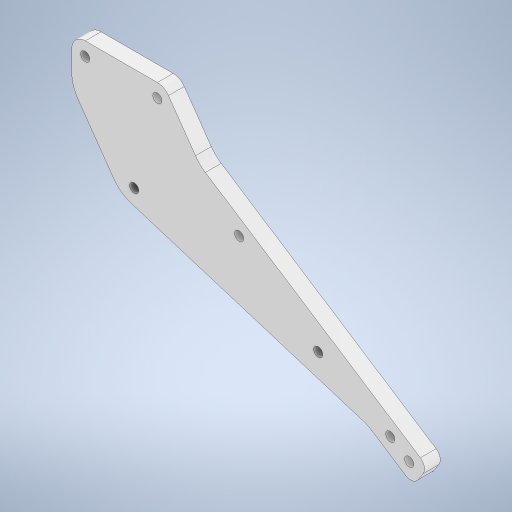
# Autodesk Inventor part: Tibia_V2
Saved by Autodesk Inventor 2024 (Build 280153000, 153)
## iProperties
Created: 2024-06-04
Part Number: Tibia_V2
Material: Generic
Document SubType Name: Modeling
Designer: Hemant
Density: 1 g/cm^3
Appearance: White
Author: Hemant
Autodesk Inventor part; units mm, degrees
ref_plane "YZ Plane" through (0, 0, 0) normal (1, 0, 0) x (0, 1, 0)
ref_plane "XZ Plane" through (0, 0, 0) normal (0, 1, 0) x (-1, 0, 0)
ref_plane "XY Plane" through (0, 0, 0) normal (0, 0, 1) x (1, 0, 0)
sketch "Sketch1" plane through (0, 0, 0) normal (0, 0, 1) x (1, 0, 0)
  line L0 (0, 0) -> (22, 0)
  circle A0 centre (3, -3) radius 1
  circle A1 centre (19, -3) radius 1
  circle A2 centre (19, -3) radius 3
  circle A3 centre (3, -3) radius 3
  line L1 (0, -10) -> (27.5638, -10) construction
  line L2 (22, 0) -> (30.0637, -11.5162) construction
  line L3 (22, 0) -> (36.0586, 0) construction
  line L4 (0, -10) -> (0, -3)
  line L5 (28.3404, -11.1091) -> (21.4575, -1.2793)
  line L6 (0, -10) -> (10.7416, -25.3406)
  circle A4 centre (26.0021, -13) radius 1 construction
  line L7 (28.3404, -11.1091) -> (79, -44.0078)
  line L8 (28.3404, -11.1091) -> (26.0021, -13) construction
  line L9 (26.0021, -13) -> (10.7416, -25.3406) construction
  circle A5 centre (13.8594, -22.8194) radius 1
  line L10 (79, -101.0698) -> (79, 42.0759) construction
  line L11 (79, -44.0078) -> (75.7322, -49.0399)
  circle A6 centre (74.8501, -44.8899) radius 1
  line L12 (75.7322, -49.0399) -> (65.6681, -42.5042)
  circle A7 centre (70.6567, -42.1667) radius 1
  line L13 (65.6681, -42.5042) -> (10.7416, -25.3406)
  circle A8 centre (13.8594, -22.8194) radius 3 construction
  circle A9 centre (26.0021, -13) radius 3 construction
  line L14 (67.4577, -36.7773) -> (-2.3075, -14.9769) construction
  line L15 (-2.3075, -14.9769) -> (-9.5668, -6) construction
  line L16 (90.7322, -58.781) -> (24.0944, -15.5059) construction
  line L17 (24.0944, -15.5059) -> (16.5425, -4.7207) construction
  line L18 (47.0108, -30.388) -> (1.9372, -16.3033) construction
  line L19 (1.9372, -16.3033) -> (12.3526, -7.8807) construction
  line L20 (12.3526, -7.8807) -> (47.0108, -30.388) construction
  line L21 (0, -6) -> (22, -6) construction
  line L22 (-9.5668, -6) -> (17.4383, -6) construction
  line L23 (17.4383, -6) -> (22.4483, -13.155) construction
  line L24 (22.4483, -13.155) -> (6.5898, -25.9792) construction
  line L25 (6.5898, -25.9792) -> (-9.5668, -6) construction
  circle A10 centre (54.6727, -33.8896) radius 1
  circle A11 centre (37.1374, -20.399) radius 1
  circle A12 centre (37.1374, -20.399) radius 3 construction
  point P0 (19, 0)
  point P1 (3, 0)
  dimension "d0" = 22
  dimension "d1" = 2
  dimension "d2" = 2
  dimension "d3" = 16
  dimension "d4" = 3
  dimension "d5" = 3
  dimension "d6" = 2
  dimension "d7" = 2
  dimension "d8" = 10
  dimension "d9" = 55
  dimension "d10" = 2
  dimension "d11" = 13
  dimension "d12" = 3
  dimension "d13" = 158
  dimension "d14" = 2
  dimension "d15" = 4
  dimension "d17" = 60
  dimension "d19" = 2
  dimension "d20" = 6
  dimension "d21" = 3
  dimension "d22" = 3
  dimension "d23" = 12
  dimension "d24" = 6
  dimension "d25" = 2
  dimension "d26" = 5
  dimension "d27" = 12
  dimension "d28" = 3
  dimension "d29" = 2
  dimension "d30" = 2
  dimension "d31" = 6
  dimension "d32" = 6
  dimension "d33" = 6
  dimension "d40" = 2
  dimension "d41" = 18
  dimension "d42" = 2
  dimension "d43" = 6
  constraints: 52 end point, 14 point on line, 11 centre point, 7 parallel, 3 vertical, 2 horizontal, 2 perpendicular, 1 coincident, 1 collinear, 1 equal length, 1 horizontal alignment, 1 tangent, 8 other
  measures "d0" distance of L0.start L0.end
  measures "d1" diameter of A0
  measures "d2" diameter of A1
  measures "d3" distance of A1.centre A0.centre
  measures "d4" horizontal distance of L0.start A0.centre
  measures "d5" distance from line of L0 A0.centre
  measures "d6" diameter of A1
  measures "d7" diameter of A0
  measures "d8" distance between parallel lines of L0 L1
  measures "d9" angle of L2 L3
  measures "d10" diameter of A4
  measures "d11" distance from line of L0 L8.end
  measures "d12" distance from line of L8.end L5
  measures "d13" angle of L5 L7
  measures "d14" diameter of A5
  measures "d15" distance from line of L6 A5.centre
  measures "d17" distance from line of L10 A1.centre
  measures "d19" diameter of A6
  measures "d20" distance of L7.end L11.end
  measures "d21" distance from line of L7 A6.centre
  measures "d22" distance from line of L11 A6.centre
  measures "d23" distance of L12.start L12.end
  measures "d24" distance between parallel lines of L7 L12
  measures "d25" diameter of A7
  measures "d26" distance of A7.centre A6.centre
  measures "d27" distance of L5.start L5.end
  measures "d28" distance from line of L7 A7.centre
  measures "d29" radial gap between concentric circles of A5 A8
  measures "d30" radial gap between concentric circles of A4 A9
  measures "d31" distance between parallel lines of L13 L14
  measures "d32" distance between parallel lines of L7 L16
  measures "d33" distance between parallel lines of L0 L21
  measures "d40" diameter of A10
  measures "d41" distance of A10.centre A7.centre
  measures "d42" diameter of A11
  measures "d43" diameter of A12
extrude "Extrusion1" add sketch "Sketch1" along normal blind 3.5
fillet "Fillet2" radius 8 4 edges at (10.7416, -25.3406, 1.75) (0, -10, 1.75) (28.3404, -11.1091, 1.75) (65.6681, -42.5042, 1.75)
fillet "Fillet3" radius 2 2 edges at (79, -44.0078, 1.75) (75.7322, -49.0399, 1.75)
equation "\"d24\" = d20"
body "Solid1"
